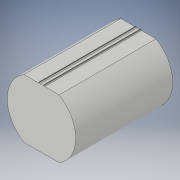
# Autodesk Inventor part: corridor
Saved by Autodesk Inventor 2017 (Build 210142000, 142)
## iProperties
Created: 2018-03-04
Part Number: corridor
Material: Generic
Document SubType Name: Modeling
Designer: Braxton
Density: 1 g/cm^3
Appearance: Default
Author: Braxton
Autodesk Inventor part; units mm, degrees
ref_plane "YZ Plane" through (0, 0, 0) normal (1, 0, 0) x (0, 1, 0)
ref_plane "XZ Plane" through (0, 0, 0) normal (0, 1, 0) x (-1, 0, 0)
ref_plane "XY Plane" through (0, 0, 0) normal (0, 0, 1) x (1, 0, 0)
sketch "Sketch1" plane through (0, 0, 0) normal (0, 0, 1) x (1, 0, 0)
  line L0 (-50.8, -84.6667) -> (50.8, -84.6667)
  arc A0 (-50.8, 84.6667) -> (-50.8, -84.6667) centre (0, 0) ccw
  arc A1 (50.8, -84.6667) -> (50.8, 84.6667) centre (0, 0) ccw
  line L1 (0, 84.67) -> (0, 87.8623) construction
  line L2 (-7.4083, 87.8623) -> (-7.4083, 86.2542)
  line L3 (7.4083, 87.8623) -> (7.4083, 86.2542)
  line L4 (8.9958, 84.6667) -> (50.8, 84.6667)
  line L5 (-8.9958, 84.6667) -> (8.9958, 84.6667) construction
  arc A2 (7.4083, 86.2542) -> (8.9958, 84.6667) centre (8.9958, 86.2542) ccw
  arc A3 (-8.9958, 84.6667) -> (-7.4083, 86.2542) centre (-8.9958, 86.2542) ccw
  line L6 (-8.9958, 84.6667) -> (-50.8, 84.6667)
  line L7 (-6.35, 87.8623) -> (-6.35, 86.6385)
  line L8 (-6.3485, 84.6873) -> (-3.1735, 87.8623) construction
  line L9 (0, 84.6667) -> (0, 87.8623) construction
  arc A4 (-3.1736, 84.6667) -> (-6.35, 87.8623) centre (-6.3485, 84.6873) ccw construction
  line L10 (4.1034, 84.6667) -> (0, 84.6667)
  line L11 (6.35, 87.8623) -> (0, 87.8623) construction
  line L12 (6.35, 87.8623) -> (6.35, 86.6385)
  line L13 (6.3485, 84.6873) -> (3.1735, 87.8623) construction
  arc A5 (6.35, 87.8623) -> (3.1736, 84.6667) centre (6.3485, 84.6873) ccw construction
  arc A6 (4.1034, 84.6667) -> (6.35, 86.6385) centre (4.1034, 86.9324) ccw
  line L14 (-6.35, 87.8623) -> (0, 87.8623) construction
  line L15 (-4.1034, 84.6667) -> (0, 84.6667)
  arc A7 (-6.35, 86.6385) -> (-4.1034, 84.6667) centre (-4.1034, 86.9324) ccw
  line L16 (7.4083, 87.8623) -> (6.35, 87.8623)
  line L17 (-6.35, 87.8623) -> (-7.4083, 87.8623)
  dimension "d1" = 101.6
  dimension "d23" = 14.8167
  dimension "d27" = 98.7374
  dimension "d28" = 98.7374
  dimension "d30" = 43.3917
  dimension "d39" = 1.5875
  dimension "d40" = 1.5875
  dimension "d41" = 41.8042
  dimension "d51" = 6.35
  dimension "d52" = 3.175
  dimension "d53" = 2.2657
  dimension "d54" = 2.2466
  dimension "d55" = 45
  dimension "d56" = 84.6667
  constraints: 36 end point, 19 point on circle, 10 symmetric about line, 8 centre point, 6 point on line, 4 collinear, 4 perpendicular, 3 coincident, 2 horizontal, 2 tangent, 1 parallel, 1 vertical, 3 other
  measures "d1" distance of L6.end L4.end
  measures "d23" distance of L2.start L3.start
  measures "d27" radius of A0
  measures "d28" radius of A1
  measures "d30" distance from line of L6.end L2
  measures "d39" distance from line of L4.start L3
  measures "d40" radius of A2
  measures "d41" distance of L4.start L4.end
  measures "d51" distance of L1.end L7.start
  measures "d52" distance of L7.start L8.start
  measures "d53" radius of A7
  measures "d54" horizontal distance of L15.start L7.end
  measures "d55" angle of L14 L8
  measures "d56" distance from line of L0 point (0, 0)
extrude "corridor" add sketch "Sketch1" along normal blind 279.4
equation "\"d28\" = d27"
equation "\"d39\" = 0.5 * d26"
equation "\"d26\" = 3.175"
body "Solid1"
